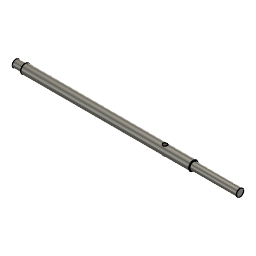
input-shaft (Autodesk Fusion 360 design; units mm, degrees)
part number: 2026-06-06-15-28-21-803
Autodesk Fusion 360 part; units mm, degrees
sketch "Sketch1" plane through (0, 0, 0) normal (1, 0, 0) x (0, 1, 0)
  circle A0 centre (0, 0) radius 5
  dimension "d1" = 10
  constraint coincident A0.centre origin
  measures "d1" diameter of A0
extrude "Extrude1" add sketch "Sketch1" along normal blind 130
sketch "Sketch2" plane through (130, 0, 0) normal (1, 0, 0) x (0, 0, -1)
  circle A0 centre (0, 0) radius 5
  circle A1 centre (0, 0) radius 4
  dimension "d4" = 8
  constraint coincident A0.centre A1.centre
  measures "d4" diameter of A1
extrude "Extrude2" cut sketch "Sketch2" against normal blind 50
sketch "Sketch3" plane through (0, 0, 0) normal (-1, 0, 0) x (0, 0, 1)
  circle A0 centre (0, 0) radius 5
  circle A1 centre (0, 0) radius 4
  dimension "d7" = 8
  constraint concentric A0 A1
  measures "d7" diameter of A1
extrude "Extrude3" cut sketch "Sketch3" against normal blind 20
extrude "Extrude4" add 1 faces at (20, 4.6443, -0.348) along direction (-1, 0, 0) blind 5
extrude "Extrude5" cut 1 faces at (0, -0.5286, 1.4202) along direction (1, 0, 0) blind 5
extrude "Extrude6" add 1 faces at (80, 4.6443, 0.348) along direction (1, 0, 0) blind 52
extrude "Extrude7" add 1 faces at (130, -0.2204, 1.0288) along direction (1, 0, 0) blind 12
extrude "Extrude8" add 1 faces at (142, -0.2204, 1.0288) along direction (1, 0, 0) blind 40
sketch "Sketch4" plane through (0, 0, 0) normal (0, 1, 0) x (1, 0, 0)
sketch "Sketch5" plane through (0, 0, 0) normal (0, 1, 0) x (1, 0, 0)
sketch "Sketch6" plane through (0, 0, 0) normal (0, 1, 0) x (1, 0, 0)
  line L0 (132, 0) -> (107, 0)
  circle A0 centre (107, 0) radius 2.25
  dimension "d20" = 25
  dimension "d21" = 4.5
  constraint horizontal L0
  constraint coincident L0.end A0.centre
  measures "d20" distance of L0.start L0.end
  measures "d21" diameter of A0
sketch "Sketch7" plane through (0, 0, 0) normal (0, 1, 0) x (1, 0, 0)
  line L0 (107, 0) -> (85, 0)
  constraint horizontal L0
sketch "Sketch9" plane through (0, 0, 0) normal (0, 1, 0) x (1, 0, 0)
  circle A0 centre (102, 0) radius 2.25
  line L0 (132, -5) -> (132, 5)
  dimension "d32" = 4.5
  dimension "d33" = 30
  measures "d32" diameter of A0
  measures "d33" distance of A0.centre L0
extrude "Extrude13" cut sketch "Sketch9" along normal mid plane 20
sketch "Sketch10" plane through (0, 0, 0) normal (0, 1, 0) x (1, 0, 0)
extrude "Extrude14" add 1 faces at (5, -0.5286, 1.4202) along direction (-1, 0, 0) blind 63
extrude "Extrude15" add 1 faces at (15, 4.6443, -0.348) along direction (-1, 0, 0) blind 63
sketch "Sketch8" plane through (0, 0, 0) normal (0, 1, 0) x (1, 0, 0)
extrude "Extrude11" [suppressed]
extrude "Extrude12" [suppressed]
